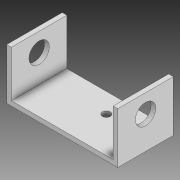
# Autodesk Inventor part: CamMount
Saved by Autodesk Inventor 2020 (Build 240168000, 168)
## iProperties
Created: 2021-03-19
Part Number: CamMount
Material: Generic
Document SubType Name: Modeling
Designer: DDeGo
Density: 1 g/cm^3
Appearance: Default
Author: DDeGo
Autodesk Inventor part; units mm, degrees
ref_plane "YZ Plane" through (0, 0, 0) normal (1, 0, 0) x (0, 1, 0)
ref_plane "XZ Plane" through (0, 0, 0) normal (0, 1, 0) x (-1, 0, 0)
ref_plane "XY Plane" through (0, 0, 0) normal (0, 0, 1) x (1, 0, 0)
sketch "Sketch1" plane through (0, 0, 0) normal (0, 0, 1) x (1, 0, 0)
  line L0 (0, 0) -> (0, 55)
  line L1 (0, 55) -> (5, 55)
  line L2 (5, 55) -> (5, 5)
  line L3 (5, 5) -> (115, 5)
  line L4 (115, 5) -> (115, 55)
  line L5 (115, 55) -> (120, 55)
  line L6 (120, 55) -> (120, 0)
  line L7 (120, 0) -> (0, 0)
  dimension "d0" = 5
  dimension "d1" = 50
  dimension "d2" = 120
  dimension "d3" = 5
  constraints: 16 end point, 6 perpendicular, 2 point on line, 1 collinear, 1 vertical
  measures "d0" distance between parallel lines of L0 L2
  measures "d1" distance of L1.end L2.end
  measures "d2" distance between parallel lines of L6 L0
  measures "d3" distance between parallel lines of L7 L3
extrude "Extrusion1" add sketch "Sketch1" along normal blind 60
sketch "Sketch2" plane through (120, 0, 0) normal (1, 0, 0) x (0, 0, -1)
  line L0 (0, 55) -> (-60, 55) projected
  line L1 (-30, 55) -> (-30, 35) construction
  circle A0 centre (-30, 35) radius 11
  point P0 (0, 0)
  dimension "d6" = 22
  dimension "d7" = 20
  constraints: 2 end point, 1 centre point, 1 coincident, 1 midpoint, 1 vertical
  measures "d6" diameter of A0
  measures "d7" distance of L1.start L1.end
extrude "Extrusion2" cut sketch "Sketch2" against normal through all
sketch "Sketch3" plane through (5, 5, 0) normal (0, 1, 0) x (1, 0, 0)
  circle A0 centre (64.0144, -21.3023) radius 4.2811
  point P0 (-5, 0)
  constraints: 1 centre point
extrude "Extrusion3" cut sketch "Sketch3" against normal through all
body "Solid1"
